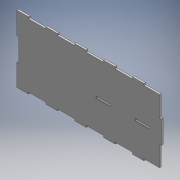
# Autodesk Inventor part: latOpSupp
Saved by Autodesk Inventor 2016 (Build 200138000, 138)
## iProperties
Created: 2016-12-12
Part Number: latOpSupp
Material: Generic
Document SubType Name: Modeling
Designer: NacostaMobile
Density: 1 g/cm^3
Appearance: Default
Author: NacostaMobile
Autodesk Inventor part; units mm, degrees
ref_plane "YZ Plane" through (0, 0, 0) normal (1, 0, 0) x (0, 1, 0)
ref_plane "XZ Plane" through (0, 0, 0) normal (0, 1, 0) x (-1, 0, 0)
ref_plane "XY Plane" through (0, 0, 0) normal (0, 0, 1) x (1, 0, 0)
sketch "Sketch1" plane through (0, 0, 0) normal (0, 1, 0) x (-1, 0, 0)
  line L0 (0, 0) -> (0, -3)
  line L1 (-250, -38) -> (-250, -78)
  line L2 (0, 0) -> (-20, 0)
  line L3 (-50, 0) -> (-50, -3)
  line L4 (-50, 0) -> (-70, 0)
  line L5 (-70, 0) -> (-70, -3)
  line L6 (-100, 0) -> (-100, -3)
  line L7 (-100, 0) -> (-120, 0)
  line L8 (-120, 0) -> (-120, -3)
  line L9 (-150, 0) -> (-150, -3)
  line L10 (-150, 0) -> (-170, 0)
  line L11 (-170, 0) -> (-170, -3)
  line L12 (-200, 0) -> (-200, -3)
  line L13 (-200, 0) -> (-220, 0)
  line L14 (-220, 0) -> (-220, -3)
  line L15 (-20, 0) -> (-20, -3)
  line L16 (-250, -58) -> (-250, -78)
  line L17 (-250, -78) -> (-247, -78)
  line L18 (-247, -78) -> (-247, -113)
  line L19 (-250, -58) -> (-250, -38)
  line L20 (-250, -38) -> (-247, -38)
  line L21 (-247, -38) -> (-247, -3)
  line L22 (-220, -3) -> (-247, -3)
  line L23 (-170, -3) -> (-200, -3)
  line L24 (-120, -3) -> (-150, -3)
  line L25 (-20, -3) -> (-50, -3)
  line L26 (-70, -3) -> (-100, -3)
  line L27 (0, -116) -> (0, -113)
  line L28 (0, -116) -> (-20, -116)
  line L29 (-50, -116) -> (-50, -113)
  line L30 (-50, -116) -> (-70, -116)
  line L31 (-70, -116) -> (-70, -113)
  line L32 (-100, -116) -> (-100, -113)
  line L33 (-100, -116) -> (-120, -116)
  line L34 (-120, -116) -> (-120, -113)
  line L35 (-150, -116) -> (-150, -113)
  line L36 (-150, -116) -> (-170, -116)
  line L37 (-170, -116) -> (-170, -113)
  line L38 (-200, -116) -> (-200, -113)
  line L39 (-200, -116) -> (-220, -116)
  line L40 (-220, -116) -> (-220, -113)
  line L41 (-20, -116) -> (-20, -113)
  line L42 (-3, -58) -> (-3, -78)
  line L43 (-3, -78) -> (0, -78)
  line L44 (-3, -58) -> (-3, -38)
  line L45 (-3, -38) -> (0, -38)
  line L46 (0, -113) -> (0, -78)
  line L47 (0, -38) -> (0, -3)
  line L48 (-50, -113) -> (-20, -113)
  line L49 (-100, -113) -> (-70, -113)
  line L50 (-150, -113) -> (-120, -113)
  line L51 (-247, -113) -> (-220, -113)
  line L52 (-200, -113) -> (-170, -113)
  line L53 (-230, -60) -> (-205, -60)
  line L54 (-205, -60) -> (-205, -63)
  line L55 (-205, -63) -> (-230, -63)
  line L56 (-230, -63) -> (-230, -60)
  line L57 (-162, -60) -> (-137, -60)
  line L58 (-137, -60) -> (-137, -63)
  line L59 (-137, -63) -> (-162, -63)
  line L60 (-162, -63) -> (-162, -60)
  dimension "d2" = 110
  dimension "d3" = 20
  dimension "d4" = 20
  dimension "d5" = 20
  dimension "d7" = 20
  dimension "d8" = 20
  dimension "d9" = 20
  dimension "d10" = 3
  dimension "d11" = 20
  dimension "d12" = 3
  dimension "d13" = 250
  dimension "d14" = 30
  dimension "d15" = 30
  dimension "d16" = 30
  dimension "d17" = 30
  dimension "d23" = 25
  dimension "d24" = 3
  dimension "d25" = 43
  dimension "d26" = 25
  dimension "d27" = 3
  dimension "d28" = 57
  dimension "d31" = 17
  dimension "d32" = 2
  dimension "d33" = 3
  dimension "d34" = 40
  dimension "d35" = 110
  constraints: 122 end point, 77 perpendicular, 8 point on line, 6 parallel, 3 vertical, 1 horizontal, 1 midpoint
  measures "d2" distance of L21.end L18.end
  measures "d3" distance of L0.start L2.end
  measures "d4" distance of L3.start L4.end
  measures "d5" distance of L6.start L7.end
  measures "d7" distance of L9.start L10.end
  measures "d8" distance of L12.start L13.end
  measures "d9" distance of L1.end L16.start
  measures "d10" distance of L1.end L17.end
  measures "d11" distance of L1.start L16.start
  measures "d12" distance of L1.start L20.end
  measures "d13" distance between parallel lines of L46 L1
  measures "d14" distance of L15.end L3.end
  measures "d15" distance of L5.end L6.end
  measures "d16" distance of L8.end L9.end
  measures "d17" distance of L11.end L12.end
  measures "d23" distance of L53.start L53.end
  measures "d24" distance of L53.end L54.end
  measures "d25" distance of L53.end L57.start
  measures "d26" distance of L57.start L57.end
  measures "d27" distance of L57.end L58.end
  measures "d28" distance between parallel lines of L57 L23
  measures "d31" distance between parallel lines of L56 L18
  measures "d32" distance from line of L16.start L53
  measures "d33" distance between parallel lines of L47 L44
  measures "d34" distance between parallel lines of L43 L45
  measures "d35" distance from line of L18 L58.end
extrude "Extrusion2" add sketch "Sketch1" along normal blind 3
body "Solid2"
